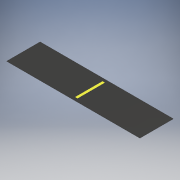
# Autodesk Inventor part: black_mid_empty
Saved by Autodesk Inventor 2019 (Build 230136000, 136)
## iProperties
Created: 2020-04-29
Part Number: black_mid_empty
Material: Generic
Document SubType Name: Modeling
Designer: infinity
Density: 1 g/cm^3
Appearance: Smooth - Black
Author: infinity
Autodesk Inventor part; units mm, degrees
ref_plane "YZ Plane" through (0, 0, 0) normal (1, 0, 0) x (0, 1, 0)
ref_plane "XZ Plane" through (0, 0, 0) normal (0, 1, 0) x (-1, 0, 0)
ref_plane "XY Plane" through (0, 0, 0) normal (0, 0, 1) x (1, 0, 0)
sketch "Sketch1" plane through (0, 0, 0) normal (0, 1, 0) x (-1, 0, 0)
  line L0 (0, 0) -> (1219.2, 0)
  line L1 (1219.2, 0) -> (1219.2, -304.8)
  line L2 (1219.2, -304.8) -> (0, -304.8)
  line L3 (0, -304.8) -> (0, 0)
  dimension "d0" = 1219.2
  dimension "d1" = 304.8
  constraints: 8 end point, 2 parallel, 1 horizontal, 1 perpendicular
  measures "d0" distance of L1.end L2.end
  measures "d1" distance of L0.end L1.end
extrude "Extrusion1" add sketch "Sketch1" along normal blind 2.54
sketch "Sketch2" plane through (0, 2.54, 0) normal (0, 1, 0) x (1, 0, 0)
  line L0 (-622.3, 279.4) -> (-596.9, 279.4)
  line L1 (-596.9, 279.4) -> (-596.9, 25.4)
  line L2 (-596.9, 25.4) -> (-622.3, 25.4)
  line L3 (-622.3, 25.4) -> (-622.3, 279.4)
  line L4 (-609.6, 791.1574) -> (-609.6, -567.1744) construction
  line L5 (0, 0) -> (0, 304.8) projected
  line L6 (0, 304.8) -> (-1219.2, 304.8) projected
  dimension "d4" = 254
  dimension "d5" = 25.4
  dimension "d6" = 609.6
  dimension "d7" = 12.7
  dimension "d8" = 25.4
  constraints: 10 end point, 2 parallel, 1 horizontal, 1 perpendicular, 1 vertical
  measures "d4" distance of L0.end L1.end
  measures "d5" distance of L0.start L0.end
  measures "d6" distance between parallel lines of L5 L4
  measures "d7" distance between parallel lines of L4 L3
  measures "d8" distance between parallel lines of L6 L0
extrude "Extrusion2" add sketch "Sketch2" along normal blind 0.254
equation "\"d7\" = 0.5 * d5"
equation "\"d8\" = d5"
body "Solid1"
